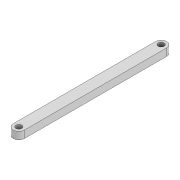
# Autodesk Inventor part: Part_4
Saved by Autodesk Inventor 2022 (Build 260153000, 153)
## iProperties
Created: 2022-04-22
Part Number: Part_4
Material: Generic
Document SubType Name: Modeling
Designer: dell
Density: 1 g/cm^3
Appearance: Default
Author: dell
Autodesk Inventor part; units mm, degrees
ref_plane "YZ Plane" through (0, 0, 0) normal (1, 0, 0) x (0, 1, 0)
ref_plane "XZ Plane" through (0, 0, 0) normal (0, 1, 0) x (-1, 0, 0)
ref_plane "XY Plane" through (0, 0, 0) normal (0, 0, 1) x (1, 0, 0)
sketch "Sketch1" plane through (0, 0, 0) normal (0, 1, 0) x (-1, 0, 0)
  line L0 (0, 0) -> (0, -76.957) construction
  line L1 (3, 0) -> (3, -76.957)
  line L2 (-3, -76.957) -> (-3, 0)
  arc A0 (3, 0) -> (-3, 0) centre (0, 0) ccw
  arc A1 (-3, -76.957) -> (3, -76.957) centre (0, -76.957) ccw
  circle A2 centre (0, 0) radius 1.6
  circle A3 centre (0, -76.957) radius 1.6
  point P0 (0, -38.4785)
  dimension "d0" = 3.2
  dimension "d1" = 3.2
  dimension "d2" = 6
  dimension "d3" = 76.957
  constraints: 8 end point, 4 centre point, 4 point on circle, 4 tangent, 2 coincident, 1 midpoint, 1 parallel, 1 vertical
  measures "d0" diameter of A2
  measures "d1" diameter of A3
  measures "d2" distance between parallel lines of L2 L1
  measures "d3" distance of L0.end L0.start
extrude "Extrusion1" add sketch "Sketch1" along normal blind 4
body "Solid1"
